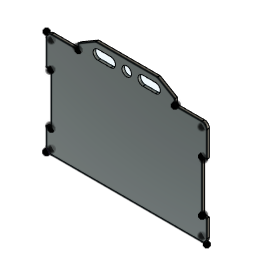
CW-NameTag (Autodesk Fusion 360 design; units mm, degrees)
Autodesk Fusion 360 part; units mm, degrees
sketch "Skizze5" plane through (0, 0, 0) normal (0, 1, 0) x (1, 0, 0)
  line L0 (3, 0) -> (97, 0)
  line L1 (80, -66) -> (80, -68.7)
  line L2 (69.2, -75) -> (30.8, -75)
  line L3 (20, -68.7) -> (20, -66)
  line L4 (97, -65) -> (81, -65)
  line L5 (19, -65) -> (3, -65)
  line L6 (20, -68.7) -> (30.8, -75)
  line L7 (80, -68.7) -> (69.2, -75)
  arc A0 (20, -66) -> (19, -65) centre (19, -66) ccw
  arc A1 (81, -65) -> (80, -66) centre (81, -66) ccw
  arc A2 (0, -62) -> (3, -65) centre (3, -62) ccw
  arc A3 (97, -65) -> (100, -62) centre (97, -62) ccw
  arc A4 (100, -3) -> (97, 0) centre (97, -3) ccw
  arc A5 (3, 0) -> (0, -3) centre (3, -3) ccw
  line L8 (0, -46) -> (2, -46)
  line L9 (3, -45) -> (3, -15)
  line L10 (2, -14) -> (0, -14)
  line L11 (0, -62) -> (0, -46)
  line L12 (0, -14) -> (0, -3)
  arc A6 (2, -46) -> (3, -45) centre (2, -45) ccw
  arc A7 (3, -15) -> (2, -14) centre (2, -15) ccw
  line L13 (100, -46) -> (98, -46)
  line L14 (97, -45) -> (97, -15)
  line L15 (98, -14) -> (100, -14)
  line L16 (100, -3) -> (100, -14)
  line L17 (100, -46) -> (100, -62)
  arc A8 (97, -45) -> (98, -46) centre (98, -45) ccw
  arc A9 (98, -14) -> (97, -15) centre (98, -15) ccw
  point P0 (100, 0)
  point P1 (0, -65)
  point P2 (20, -65)
  point P3 (80, -65)
  point P4 (3, -46)
  point P5 (3, -14)
  point P6 (97, -46)
  point P7 (97, -14)
  dimension "d46" = 100
  dimension "d47" = 65
  dimension "d48" = 20
  dimension "d49" = 20
  dimension "d51" = 3.7
  dimension "d52" = 3.7
  dimension "d53" = 10.8
  dimension "d54" = 10.8
  dimension "d55" = 10
  dimension "d56" = 1
  dimension "d57" = 1
  dimension "d58" = 3
  dimension "d59" = 3
  dimension "d60" = 3
  dimension "d61" = 3
  dimension "d62" = 3
  dimension "d63" = 32
  dimension "d64" = 14
  dimension "d65" = 1
  dimension "d66" = 1
  dimension "d67" = 32
  dimension "d68" = 14
  dimension "d69" = 3
  dimension "d70" = 1
  dimension "d71" = 1
  constraint horizontal L0
  constraint vertical L16
  constraint horizontal L4
  constraint vertical L11
  constraint vertical L1
  constraint horizontal L2
  constraint vertical L3
  constraint coincident P2 L4
  constraint collinear L4 L5
  constraint coincident P2 L3
  constraint coincident P2 L5
  constraint tangent L3 A0
  constraint tangent L5 A0
  constraint coincident P3 L1
  constraint coincident P3 L4
  constraint tangent L1 A1
  constraint tangent L4 A1
  constraint coincident P1 L11
  constraint coincident P1 L5
  constraint tangent A2 L11
  constraint tangent L5 A2
  constraint tangent A3 L16
  constraint tangent L4 A3
  constraint coincident P0 L0
  constraint coincident P0 L16
  constraint tangent L0 A4
  constraint tangent A4 L16
  constraint coincident origin L0
  constraint coincident origin L11
  constraint tangent L0 A5
  constraint tangent A5 L11
  constraint horizontal L8
  constraint vertical L9
  constraint horizontal L10
  constraint coincident L10.end L11
  constraint collinear L11 L12
  constraint coincident P4 L8
  constraint coincident P4 L9
  constraint tangent L8 A6
  constraint tangent L9 A6
  constraint coincident P5 L9
  constraint coincident P5 L10
  constraint tangent L9 A7
  constraint tangent L10 A7
  constraint horizontal L13
  constraint vertical L14
  constraint horizontal L15
  constraint coincident L13.start L16
  constraint collinear L16 L17
  constraint coincident P6 L13
  constraint coincident P6 L14
  constraint tangent L13 A8
  constraint tangent L14 A8
  constraint coincident P7 L14
  constraint coincident P7 L15
  constraint tangent L14 A9
  constraint tangent L15 A9
  measures "d46" distance of origin P0
  measures "d47" distance of origin P1
  measures "d48" distance of L3 L11
  measures "d49" distance of L1 L16
  measures "d51" distance of L5 L3.start
  measures "d52" distance of L4 L1.end
  measures "d53" horizontal distance of P3 L2.start
  measures "d54" horizontal distance of P2 L2.end
  measures "d55" distance of L2 L4
  measures "d56" radius of A0
  measures "d57" radius of A1
  measures "d58" radius of A2
  measures "d59" radius of A3
  measures "d60" radius of A4
  measures "d61" radius of A5
  measures "d62" distance of L9 L11
  measures "d63" distance of P4 P5
  measures "d64" distance of L0 L10
  measures "d65" radius of A6
  measures "d66" radius of A7
  measures "d67" distance of P6 P7
  measures "d68" distance of L0 L15
  measures "d69" distance of L14 L16
  measures "d70" radius of A8
  measures "d71" radius of A9
extrude "Extrusion1" add sketch "Skizze5" along normal blind 1.6
sketch "Skizze6" plane through (0, 0, 0) normal (0, -1, 0) x (1, 0, 0)
  arc A0 (97, 0) -> (100, 3) centre (97, 3) ccw
  line L0 (100, 3) -> (100, 14)
  line L1 (100, 14) -> (98, 14)
  arc A1 (97, 15) -> (98, 14) centre (98, 15) ccw
  line L2 (97, 15) -> (97, 45)
  arc A2 (98, 46) -> (97, 45) centre (98, 45) ccw
  line L3 (98, 46) -> (100, 46)
  line L4 (100, 46) -> (100, 62)
  arc A3 (100, 62) -> (97, 65) centre (97, 62) ccw
  line L5 (97, 65) -> (81, 65)
  arc A4 (80, 66) -> (81, 65) centre (81, 66) ccw
  line L6 (80, 66) -> (80, 68.7)
  line L7 (80, 68.7) -> (69.2, 75)
  line L8 (69.2, 75) -> (30.8, 75)
  line L9 (30.8, 75) -> (20, 68.7)
  line L10 (20, 68.7) -> (20, 66)
  arc A5 (19, 65) -> (20, 66) centre (19, 66) ccw
  line L11 (19, 65) -> (3, 65)
  arc A6 (3, 65) -> (0, 62) centre (3, 62) ccw
  line L12 (0, 62) -> (0, 46)
  line L13 (0, 46) -> (2, 46)
  arc A7 (3, 45) -> (2, 46) centre (2, 45) ccw
  line L14 (3, 45) -> (3, 15)
  arc A8 (2, 14) -> (3, 15) centre (2, 15) ccw
  line L15 (2, 14) -> (0, 14)
  line L16 (0, 14) -> (0, 3)
  arc A9 (0, 3) -> (3, 0) centre (3, 3) ccw
  line L17 (3, 0) -> (97, 0)
  circle A10 centre (50, 68.5) radius 3
  line L18 (32, 65.5) -> (40, 65.5)
  arc A11 (40, 65.5) -> (40, 71.5) centre (40, 68.5) ccw
  line L19 (40, 71.5) -> (32, 71.5)
  arc A12 (32, 71.5) -> (32, 65.5) centre (32, 68.5) ccw
  line L20 (32, 68.5) -> (40, 68.5) construction
  line L21 (68, 71.5) -> (60, 71.5)
  arc A13 (60, 71.5) -> (60, 65.5) centre (60, 68.5) ccw
  line L22 (60, 65.5) -> (68, 65.5)
  arc A14 (68, 65.5) -> (68, 71.5) centre (68, 68.5) ccw
  line L23 (68, 68.5) -> (60, 68.5) construction
  point P0 (36, 68.5)
  point P1 (64, 68.5)
  dimension "d77" = 50
  dimension "d78" = 68.5
  dimension "d79" = 6
  dimension "d88" = 8
  dimension "d89" = 8
  dimension "d90" = 6
  dimension "d91" = 6
  dimension "d92" = 68.5
  dimension "d93" = 68.5
  dimension "d94" = 36
  dimension "d95" = 36
  constraint tangent L18 A11
  constraint tangent A11 L19
  constraint parallel L18 L19
  constraint tangent L19 A12
  constraint tangent L18 A12
  constraint horizontal L20
  constraint midpoint L20 P0
  constraint tangent L21 A13
  constraint tangent A13 L22
  constraint parallel L21 L22
  constraint tangent L22 A14
  constraint tangent L21 A14
  constraint horizontal L23
  constraint midpoint L23 P1
  measures "d77" distance of L12 A10.centre
  measures "d78" distance of L17 A10.centre
  measures "d79" diameter of A10
  measures "d88" distance of L18.start L18.end
  measures "d89" distance of A13.end L22.end
  measures "d90" distance of L21 L22
  measures "d91" distance of L18 L19
  measures "d92" distance of L17 P1
  measures "d93" distance of L17 P0
  measures "d94" distance of L12 P0
  measures "d95" distance of L4 P1
extrude "Extrusion5" cut sketch "Skizze6" against normal blind 1.6 contours A10 | L18 A11 L19 A12 | L21 A13 L22 A14
